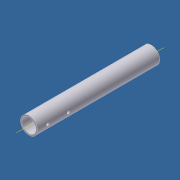
# Autodesk Inventor part: FE-00006-02
Saved by Autodesk Inventor 2012 (Build 160160000, 160)
## iProperties
Created: 2008-05-24
Part Number: FE-00006-02
Document SubType Name: Modeling
Designer: firstuser
Density: 1 g/cm^3
Mass: 129.738 g
Surface Area: 738.578 cm^2
Volume: 129.738 cm^3
Material: Default
Author: firstuser
Autodesk Inventor part; units mm, degrees
ref_plane "XZ Plane" through (0, 0, 0) normal (0, 1, 0) x (-1, 0, 0)
ref_plane "XY Plane" through (0, 0, 0) normal (0, 0, 1) x (1, 0, 0)
sketch "Sketch1" plane through (0, 0, 0) normal (0, 0, 1) x (1, 0, 0)
  circle A0 centre (0, 0) radius 21.0312
  circle A1 centre (0, 0) radius 17.4625
  dimension "d0" = 42.0624
  dimension "d1" = 34.925
  constraints: 2 centre point, 1 coincident
  measures "d0" diameter of A0
  measures "d1" diameter of A1
extrude "Extrusion1" add sketch "Sketch1" along normal blind 301.625
ref_plane "Work Plane1" through (0, 0, 0) normal (1, 0, 0) x (0, 0, 1)
sketch "Sketch2" plane through (0, 0, 0) normal (1, 0, 0) x (0, 0, 1)
  line L0 (0, -21.0312) -> (301.625, -21.0312) projected
  line L1 (0, 21.0312) -> (301.625, 21.0312) projected
  line L2 (301.625, 17.4625) -> (301.625, -17.4625) projected
  line L3 (301.625, 21.0312) -> (301.625, -21.0312) projected
  line L4 (-60.325, 0) -> (361.95, 0) projected
  circle A0 centre (276.225, 0) radius 3.175
  dimension "d5" = 25.4
  dimension "d6" = 6.35
  constraints: 1 centre point, 1 point on line
  measures "d5" distance from line of A0.centre L3
  measures "d6" diameter of A0
extrude "Extrusion2" cut sketch "Sketch2" along normal blind 50.8
pattern_linear "Rectangular Pattern1" count 2 spacing 50.8 along (0, 0, -1) of "Extrusion2"
body "Solid1"
